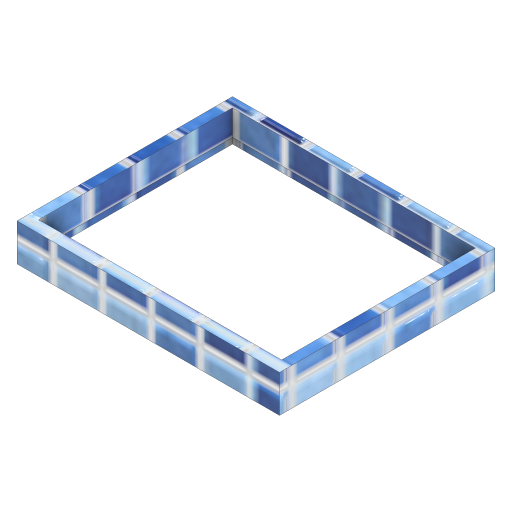
# Autodesk Inventor part: che
Saved by Autodesk Inventor 2024.3 (Build 283343000, 343)
## iProperties
Created: 2025-09-02
Part Number: che
Material: Generic
Document SubType Name: Modeling
Designer: danie
Density: 1 g/cm^3
Appearance: 1in Squares - Mosaic Blue
Author: danie
Autodesk Inventor part; units mm, degrees
ref_plane "YZ Plane" through (0, 0, 0) normal (1, 0, 0) x (0, 1, 0)
ref_plane "XZ Plane" through (0, 0, 0) normal (0, 1, 0) x (-1, 0, 0)
ref_plane "XY Plane" through (0, 0, 0) normal (0, 0, 1) x (1, 0, 0)
sketch "Sketch1" plane through (0, 0, 0) normal (0, 1, 0) x (-1, 0, 0)
  line L0 (0, 0) -> (130, 0)
  line L1 (130, 0) -> (130, -106)
  line L2 (130, -106) -> (0, -106)
  line L3 (0, -106) -> (0, 0)
  line L4 (130, 0) -> (130, -3)
  line L5 (127, -4.0545) -> (0, -4.0545)
  line L6 (0, -4.0545) -> (3, -4.0545)
  line L7 (3, -4.0545) -> (3, -106)
  line L8 (3, -106) -> (3, -103)
  line L9 (3, -103) -> (3, -101.9174)
  line L10 (3, -103) -> (130, -103)
  line L11 (130, -3) -> (127, -4.0545)
  line L12 (130, -103) -> (127, -103)
  line L13 (127, -103) -> (127, -4.0545)
  line L14 (127, -4.0545) -> (0, -4.0545)
  line L15 (0, 0) -> (0, -106)
  line L16 (0, -106) -> (130, -106)
  line L17 (130, -106) -> (130, 0)
  line L18 (127, -4.0545) -> (127, -103)
  line L19 (127, -103) -> (3, -103)
  line L20 (3, -103) -> (3, -4.0545)
  line L21 (3, -4.0545) -> (127, -4.0545)
  dimension "d0" = 130
  dimension "d1" = 106
  dimension "d2" = 3
  dimension "d3" = 3
  dimension "d4" = 3
  dimension "d5" = 3
  constraints: 44 end point, 7 point on line, 6 collinear, 6 perpendicular, 3 parallel, 1 horizontal
  measures "d0" distance of L1.end L2.end
  measures "d1" distance of L0.end L1.end
  measures "d2" distance of L0.end L4.end
  measures "d3" distance of L5.end L6.end
  measures "d4" distance of L7.end L8.end
  measures "d5" distance of L10.end L12.end
sketch "Sketch2" plane through (0, 0, 0) normal (0, 1, 0) x (-1, 0, 0)
  point P0 (0, 0)
extrude "Extrusion1" add sketch "Sketch1" along normal blind 13 contours L0 L1 L11 L5 L3 | L5 L7 L2 L3 | L1 L10 L13 L11 | L1 L2 L7 L10
sketch "Sketch6" plane through (-130, 0, 0) normal (0, 0, 1) x (1, 0, 0)
  line L0 (0, 13) -> (130, 13) projected
  line L1 (0, 13) -> (130, 13)
  line L2 (130, 13) -> (130, 0)
  line L3 (130, 0) -> (0, 0)
  line L4 (0, 0) -> (0, 13)
  constraints: 8 end point, 3 perpendicular, 1 collinear
extrude "Extrusion3" add sketch "Sketch6" along normal blind 2
sketch "Sketch7" plane through (0, 0, 0) normal (0, -1, 0) x (1, 0, 0)
  line L0 (-130, -106) -> (-130, 2) projected
  line L1 (-130, 0) -> (0, 0)
  line L2 (0, -106) -> (0, 2) projected
  line L3 (0, 0) -> (0, 2)
  line L4 (0, 2) -> (-130, 2)
  line L5 (-130, 2) -> (-130, 0)
  point P0 (-130, 2)
  constraints: 8 end point, 3 perpendicular, 1 horizontal, 1 point on line
extrude "Extrusion4" add sketch "Sketch7" along normal blind 4
sketch "Sketch8" plane through (-130, 0, -106) normal (-1, 0, 0) x (0, 0, 1)
  line L0 (108, 13) -> (108, -4) projected
  line L1 (0, 0) -> (106, 0) projected
  line L2 (108, 13) -> (0, 13)
  line L3 (0, 13) -> (0, 0)
  line L4 (0, 0) -> (108, 0)
  line L5 (108, 0) -> (108, 13)
  constraints: 8 end point, 2 parallel, 1 horizontal, 1 perpendicular
extrude "Extrusion5" add sketch "Sketch8" along normal blind 2
sketch "Sketch9" plane through (0, 0, 0) normal (0, -1, 0) x (1, 0, 0)
  line L0 (0, -106) -> (-132, -106) projected
  line L1 (-132, -106) -> (-130, -106)
  line L2 (-130, -106) -> (-130, 2.3053)
  line L3 (-127, -4.0545) -> (-127, -103) projected
  line L4 (-130, 2.3053) -> (-132, 2.3053)
  line L5 (-132, -106) -> (-132, 2) projected
  line L6 (-132, 2.3053) -> (-132, -106)
  point P0 (0, 0)
  dimension "d20" = 2
  constraints: 8 end point, 2 perpendicular, 1 parallel, 1 point on line
  measures "d20" distance of L0.end L1.end
extrude "Extrusion6" add sketch "Sketch9" along normal blind 4
sketch "Sketch10" plane through (-132, 0, -106) normal (-1, 0, 0) x (0, 0, 1)
  line L0 (108, 13) -> (108, -4) projected
  line L1 (108, 0) -> (108, -4)
  line L2 (108, -4) -> (108.3053, -4) projected
  line L3 (108.3053, 0) -> (108.3053, -4) projected
  line L4 (108.3053, -4) -> (108.3053, 0)
  line L5 (108, 0) -> (108.3053, 0)
  line L6 (108.3053, 0) -> (108.3053, -4)
  line L7 (108.3053, -4) -> (108, -4)
  point P0 (106, 0)
  constraints: 10 end point, 3 collinear, 2 perpendicular, 1 point on line
extrude "Extrusion7" cut sketch "Sketch10" against normal blind 4
sketch "Sketch11" plane through (0, 0, -106) normal (0, 0, -1) x (-1, 0, 0)
  line L0 (0, 13) -> (132, 13) projected
  line L1 (132, 13) -> (0, 13)
  line L2 (0, 13) -> (0, 0)
  line L3 (0, 0) -> (132, 0)
  line L4 (132, 0) -> (132, 13)
  constraints: 8 end point, 2 parallel, 1 horizontal, 1 perpendicular
extrude "Extrusion8" add sketch "Sketch11" along normal blind 2
sketch "Sketch12" plane through (0, 0, 0) normal (0, -1, 0) x (1, 0, 0)
  line L0 (-132, 2) -> (-132, -106) projected
  line L1 (0, -108) -> (-132, -108) projected
  line L2 (-132, -106) -> (0, -106)
  line L3 (0, -106) -> (0, -108)
  line L4 (0, -108) -> (-132, -108)
  line L5 (-132, -108) -> (-132, -106)
  point P0 (0, 0)
  constraints: 8 end point, 2 parallel, 1 horizontal, 1 perpendicular
extrude "Extrusion9" add sketch "Sketch12" along normal blind 4
sketch "Sketch13" plane through (0, -4, 2) normal (1, 0, 0) x (0, 0, -1)
  line L0 (0, 17) -> (0, 0) projected
  line L1 (110.1979, 4) -> (0, 4)
  line L2 (0, 4) -> (0, 17)
  line L3 (0, 17) -> (110.1979, 17)
  line L4 (110.1979, 17) -> (110.1979, 4)
  point P0 (2, 4)
  point P1 (0, 4)
  constraints: 8 end point, 2 parallel, 1 horizontal, 1 perpendicular
extrude "Extrusion10" add sketch "Sketch13" along normal blind 2
sketch "Sketch14" plane through (0, 0, 0) normal (0, -1, 0) x (1, 0, 0)
  line L0 (-132, -108) -> (0, -108) projected
  line L1 (2, 2) -> (2, -108.1979) projected
  line L2 (0, -108) -> (2, -108)
  line L3 (2, -108) -> (2, 2)
  line L4 (2, 2) -> (0, 2)
  line L5 (0, 2) -> (0, -108)
  point P0 (0, 0)
  constraints: 8 end point, 2 parallel, 1 horizontal, 1 perpendicular
extrude "Extrusion11" add sketch "Sketch14" along normal blind 4
sketch "Sketch15" plane through (0, 0, 0) normal (0, -1, 0) x (1, 0, 0)
  line L0 (2, -108) -> (2, -108.1979) projected
  line L1 (2, -108.1979) -> (0, -108.1979)
  line L2 (0, -108.1979) -> (0, -108)
  line L3 (0, -108) -> (2, -108)
  line L4 (2, -108) -> (2, -108.1979)
  point P0 (0, 0)
  constraints: 8 end point, 2 parallel, 1 horizontal, 1 perpendicular
extrude "Extrusion12" cut sketch "Sketch15" against normal blind 15
sketch "Sketch16" plane through (0, 0, -108) normal (0, 0, -1) x (-1, 0, 0)
  point P0 (0, 0)
sketch "Sketch17" plane through (0, -4, 0) normal (0, -1, 0) x (1, 0, 0)
  line L0 (2, 2) -> (-132, 2)
  line L1 (-132, 2) -> (-132, -108)
  line L2 (-132, -108) -> (2, -108)
  line L3 (2, -108) -> (2, 2)
  line L4 (0, -106) -> (-130, -106) projected
  line L5 (-130, 0) -> (-130, -106) projected
  line L6 (-130, -106) -> (-130, 0)
  line L7 (-130, 0) -> (0, 0)
  line L8 (0, 0) -> (0, -106)
  line L9 (0, -106) -> (-130, -106)
  constraints: 16 end point, 4 perpendicular, 3 parallel, 1 horizontal
extrude "Extrusion13" add sketch "Sketch17" along normal blind 2
body "Solid1"
